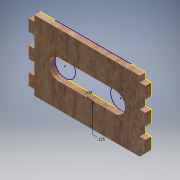
# Autodesk Inventor part: MotorShelf
Saved by Autodesk Inventor 2019 (Build 230136000, 136)
## iProperties
Created: 2019-01-17
Part Number: MotorShelf
Material: Wood (Birch)
Document SubType Name: Modeling
Designer: nxgam
Density: 0.55 g/cm^3
Appearance: Birch - Natural Polished
Mass: 14.8331 g
Surface Area: 136.304 cm^2
Volume: 26.9693 cm^3
Author: nxgam
Autodesk Inventor part; units mm, degrees
ref_plane "YZ Plane" through (0, 0, 0) normal (1, 0, 0) x (0, 1, 0)
ref_plane "XZ Plane" through (0, 0, 0) normal (0, 1, 0) x (-1, 0, 0)
ref_plane "XY Plane" through (0, 0, 0) normal (0, 0, 1) x (1, 0, 0)
sketch "Sketch1" plane through (0, 0, 0) normal (0, 0, 1) x (1, 0, 0)
  line L0 (45.72, 0) -> (45.72, 60.96)
  line L1 (45.72, 60.96) -> (-45.72, 60.96)
  line L2 (-45.72, 60.96) -> (-45.72, 9.301)
  line L3 (-45.72, 5.08) -> (-50.8, 5.08)
  line L4 (-50.8, 5.08) -> (-50.8, 15.24)
  line L5 (-50.8, 15.24) -> (-45.72, 15.24)
  line L6 (-45.72, 15.24) -> (-45.72, 5.08)
  line L7 (-45.72, 25.4) -> (-50.8, 25.4)
  line L8 (-50.8, 25.4) -> (-50.8, 35.56)
  line L9 (-50.8, 35.56) -> (-45.72, 35.56)
  line L10 (-45.72, 35.56) -> (-45.72, 25.4)
  line L11 (-45.72, 45.72) -> (-50.8, 45.72)
  line L12 (-50.8, 45.72) -> (-50.8, 55.88)
  line L13 (-50.8, 55.88) -> (-45.72, 55.88)
  line L14 (-45.72, 55.88) -> (-45.72, 45.72)
  line L15 (0, 60.96) -> (0, 0) construction
  line L16 (45.72, 60.96) -> (45.72, 0)
  line L17 (45.72, 5.08) -> (50.8, 5.08)
  line L18 (50.8, 5.08) -> (50.8, 15.24)
  line L19 (50.8, 15.24) -> (45.72, 15.24)
  line L20 (45.72, 15.24) -> (45.72, 5.08)
  line L21 (45.72, 25.4) -> (50.8, 25.4)
  line L22 (50.8, 25.4) -> (50.8, 35.56)
  line L23 (50.8, 35.56) -> (45.72, 35.56)
  line L24 (45.72, 35.56) -> (45.72, 25.4)
  line L25 (45.72, 45.72) -> (50.8, 45.72)
  line L26 (50.8, 45.72) -> (50.8, 55.88)
  line L27 (50.8, 55.88) -> (45.72, 55.88)
  line L28 (45.72, 55.88) -> (45.72, 45.72)
  line L29 (-45.72, 5.08) -> (-45.72, 0)
  line L30 (-45.72, 0) -> (45.72, 0)
  line L31 (45.72, 60.96) -> (-45.72, 60.96)
  line L32 (-45.72, 60.96) -> (-45.72, 0)
  line L33 (-45.72, 0) -> (45.72, 0)
  line L34 (45.72, 0) -> (45.72, 60.96)
  dimension "d0" = 91.44
  dimension "d2" = 10.16
  dimension "d3" = 5.08
  dimension "d7" = 20.32
  dimension "d14" = 5.08
  dimension "d15" = 60.96
  constraints: 70 end point, 12 symmetric about line, 5 parallel, 4 perpendicular, 3 vertical, 2 horizontal, 2 midpoint, 2 point on line, 1 coincident, 16 other
  measures "d0" distance of L1.end L0.end
  measures "d2" distance of L3.end L4.end
  measures "d3" distance of L4.end L5.end
  measures "d7" distance of L3.start L7.start
  measures "d14" distance of L3.start L29.end
  measures "d15" distance between parallel lines of L30 L1
extrude "Extrusion2" add sketch "Sketch1" along normal blind 5.08
sketch "Sketch5" plane through (0, 0, 5.08) normal (0, 0, 1) x (1, 0, 0)
  line L0 (50.8, 25.4) -> (50.8, 35.56) projected
  line L1 (50.8, 35.56) -> (45.72, 35.56) projected
  line L2 (45.72, 35.56) -> (45.72, 45.72) projected
  line L3 (45.72, 45.72) -> (50.8, 45.72) projected
  line L4 (50.8, 45.72) -> (50.8, 55.88) projected
  line L5 (50.8, 55.88) -> (45.72, 55.88) projected
  line L6 (45.72, 55.88) -> (45.72, 60.96) projected
  line L7 (45.72, 60.96) -> (-45.72, 60.96) projected
  line L8 (-45.72, 60.96) -> (-45.72, 55.88) projected
  line L9 (-45.72, 55.88) -> (-50.8, 55.88) projected
  line L10 (-50.8, 55.88) -> (-50.8, 45.72) projected
  line L11 (-50.8, 45.72) -> (-45.72, 45.72) projected
  line L12 (-45.72, 45.72) -> (-45.72, 35.56) projected
  line L13 (-45.72, 35.56) -> (-50.8, 35.56) projected
  line L14 (-50.8, 35.56) -> (-50.8, 25.4) projected
  line L15 (-50.8, 25.4) -> (-45.72, 25.4) projected
  line L16 (-45.72, 25.4) -> (-45.72, 15.24) projected
  line L17 (-45.72, 15.24) -> (-50.8, 15.24) projected
  line L18 (-50.8, 15.24) -> (-50.8, 5.08) projected
  line L19 (-50.8, 5.08) -> (-45.72, 5.08) projected
  line L20 (-45.72, 5.08) -> (-45.72, 0) projected
  line L21 (-45.72, 0) -> (45.72, 0) projected
  line L22 (45.72, 0) -> (45.72, 5.08) projected
  line L23 (45.72, 5.08) -> (50.8, 5.08) projected
  line L24 (50.8, 5.08) -> (50.8, 15.24) projected
  line L25 (50.8, 15.24) -> (45.72, 15.24) projected
  line L26 (45.72, 15.24) -> (45.72, 25.4) projected
  line L27 (45.72, 25.4) -> (50.8, 25.4) projected
  line L28 (-24.13, 30.48) -> (24.13, 30.48) construction
  line L29 (-24.13, 21.59) -> (24.13, 21.59)
  line L30 (24.13, 39.37) -> (-24.13, 39.37)
  arc A0 (-24.13, 39.37) -> (-24.13, 21.59) centre (-24.13, 30.48) ccw
  arc A1 (24.13, 21.59) -> (24.13, 39.37) centre (24.13, 30.48) ccw
  line L31 (45.72, 60.96) -> (-45.72, 60.96) construction
  line L32 (0, 60.96) -> (0, 0) construction
  point P0 (0, 30.48)
  dimension "d32" = 48.26
  dimension "d33" = 60.96
  dimension "d34" = 30.48
  dimension "d35" = 8.89
  constraints: 10 end point, 4 point on circle, 4 tangent, 3 midpoint, 2 centre point, 1 horizontal, 1 parallel, 1 vertical
  measures "d32" distance of L28.start L28.end
  measures "d33" distance between parallel lines of L7 L21
  measures "d34" distance between parallel lines of L21 L28
  measures "d35" radius of A1
extrude "Extrusion6" cut sketch "Sketch5" against normal blind 25.4 contours A0 L30 A1 L29
sketch "Sketch6" plane through (0, 0, 0) normal (0, 0, -1) x (-1, 0, 0)
  arc A0 (-24.13, 39.37) -> (-24.13, 21.59) centre (-24.13, 30.48) ccw projected
  line L0 (-24.13, 39.37) -> (24.13, 39.37) projected
  arc A1 (24.13, 21.59) -> (24.13, 39.37) centre (24.13, 30.48) ccw projected
  line L1 (24.13, 21.59) -> (-24.13, 21.59) projected
  line L2 (-50.8, 35.56) -> (-50.8, 25.4) projected
  line L3 (-50.8, 25.4) -> (-45.72, 25.4) projected
  line L4 (-45.72, 15.24) -> (-45.72, 25.4) projected
  line L5 (-50.8, 15.24) -> (-45.72, 15.24) projected
  line L6 (-50.8, 5.08) -> (-50.8, 15.24) projected
  line L7 (-45.72, 5.08) -> (-50.8, 5.08) projected
  line L8 (-45.72, 0) -> (-45.72, 5.08) projected
  line L9 (45.72, 0) -> (-45.72, 0) construction
  line L10 (45.72, 5.08) -> (45.72, 0) projected
  line L11 (50.8, 5.08) -> (45.72, 5.08) projected
  line L12 (50.8, 15.24) -> (50.8, 5.08) projected
  line L13 (45.72, 15.24) -> (50.8, 15.24) projected
  line L14 (45.72, 25.4) -> (45.72, 15.24) projected
  line L15 (45.72, 25.4) -> (50.8, 25.4) projected
  line L16 (50.8, 25.4) -> (50.8, 35.56) projected
  line L17 (50.8, 35.56) -> (45.72, 35.56) projected
  line L18 (45.72, 45.72) -> (45.72, 35.56) projected
  line L19 (45.72, 45.72) -> (50.8, 45.72) projected
  line L20 (50.8, 45.72) -> (50.8, 55.88) projected
  line L21 (50.8, 55.88) -> (45.72, 55.88) projected
  line L22 (45.72, 60.96) -> (45.72, 55.88) projected
  line L23 (-45.72, 60.96) -> (45.72, 60.96) projected
  line L24 (-45.72, 55.88) -> (-45.72, 60.96) projected
  line L25 (-50.8, 55.88) -> (-45.72, 55.88) projected
  line L26 (-50.8, 45.72) -> (-50.8, 55.88) projected
  line L27 (-45.72, 45.72) -> (-50.8, 45.72) projected
  line L28 (-45.72, 35.56) -> (-45.72, 45.72) projected
  line L29 (-45.72, 35.56) -> (-50.8, 35.56) projected
  line L30 (33.02, 30.48) -> (33.02, 60.96)
  line L31 (-45.72, 60.96) -> (45.72, 60.96) projected
  arc A2 (-24.13, 39.37) -> (-24.13, 21.59) centre (-24.13, 30.48) ccw projected
  line L32 (-33.02, 30.48) -> (-33.02, 60.96)
  line L33 (-33.02, 60.96) -> (33.02, 60.96)
  arc A3 (24.13, 21.59) -> (24.13, 39.37) centre (24.13, 30.48) ccw projected
  line L34 (25.8987, 21.7677) -> (0.6317, 16.6382)
  line L35 (-0.6317, 16.6382) -> (-25.8987, 21.7677)
  arc A4 (24.13, 21.59) -> (24.13, 39.37) centre (24.13, 30.48) ccw projected
  line L36 (0, 21.59) -> (0, 0) construction
  arc A5 (-0.6317, 16.6382) -> (0.6317, 16.6382) centre (0, 19.7498) ccw
  circle A6 centre (24.13, 30.48) radius 8.89
  circle A7 centre (-24.13, 30.48) radius 8.89
  point P0 (0, 16.51)
  dimension "d38" = 5.08
  dimension "d39" = 3.175
  constraints: 12 end point, 7 point on circle, 5 point on line, 5 tangent, 2 centre point, 2 coincident, 2 perpendicular, 1 collinear, 1 concentric, 1 horizontal alignment, 1 midpoint, 1 vertical, 2 other
  measures "d38" distance from line of point (0, 16.51) L1
  measures "d39" radius of A5
extrude "Extrusion7" cut sketch "Sketch6" against normal blind 25.4 contours A0 L32 L23 L30 A1 L0 | A0 L1 A1 L34 A5 L35
equation "\"d7\" = 2 * d2"
equation "\"d34\" = 0.5 * d33"
body "Solid2"
